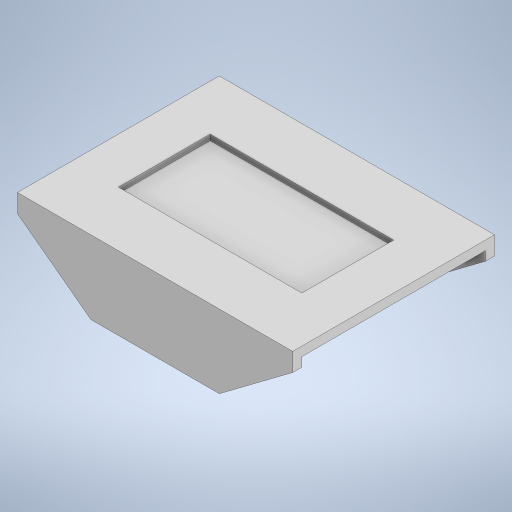
# Autodesk Inventor part: Battery Cage
Saved by Autodesk Inventor 2023 (Build 270158000, 158)
## iProperties
Created: 2022-10-27
Part Number: Battery Cage
Material: Generic
Document SubType Name: Modeling
Designer: cheng
Density: 1 g/cm^3
Appearance: Default
Author: cheng
Autodesk Inventor part; units mm, degrees
ref_plane "YZ Plane" through (0, 0, 0) normal (1, 0, 0) x (0, 1, 0)
ref_plane "XZ Plane" through (0, 0, 0) normal (0, 1, 0) x (-1, 0, 0)
ref_plane "XY Plane" through (0, 0, 0) normal (0, 0, 1) x (1, 0, 0)
sketch "Sketch1" plane through (0, 0, 0) normal (0, 1, 0) x (-1, 0, 0)
  line L0 (75, -55) -> (-75, -55)
  line L1 (-75, -55) -> (-75, 55)
  line L2 (-75, 55) -> (75, 55)
  line L3 (75, 55) -> (75, -55)
  line L4 (75, -55) -> (-75, 55) construction
  line L5 (-75, -55) -> (75, 55) construction
  point P0 (0, 0)
  dimension "d0" = 110
  dimension "d1" = 150
  constraints: 12 end point, 2 midpoint, 2 parallel, 1 horizontal, 1 perpendicular
  measures "d0" distance of L2.end L0.start
  measures "d1" distance of L0.start L0.end
extrude "Extrusion1" add sketch "Sketch1" along normal blind 40
sketch "Sketch2" plane through (75, 0, 55) normal (1, 0, 0) x (0, 0, -1)
  line L0 (55, 0) -> (55, 40)
  line L1 (105, 35) -> (5, 35)
  line L2 (5, 35) -> (5, 5)
  line L3 (5, 5) -> (105, 5)
  line L4 (105, 5) -> (105, 35)
  line L5 (105, 35) -> (5, 5) construction
  line L6 (5, 35) -> (105, 5) construction
  line L7 (0, 40) -> (110, 40) projected
  point P0 (55, 20)
  dimension "d4" = 100
  dimension "d5" = 30
  dimension "d6" = 5
  constraints: 14 end point, 3 midpoint, 2 parallel, 1 horizontal, 1 perpendicular, 1 vertical
  measures "d4" distance of L1.start L1.end
  measures "d5" distance of L3.end L1.start
  measures "d6" distance between parallel lines of L7 L1
extrude "Extrusion2" cut sketch "Sketch2" against normal through all
sketch "Sketch3" plane through (75, 0, 55) normal (1, 0, 0) x (0, 0, -1)
  line L0 (55, 0) -> (55, 5)
  line L1 (105, 5) -> (5, 5) projected
  line L2 (95, 10) -> (15, 10)
  line L3 (15, 10) -> (15, -5)
  line L4 (15, -5) -> (95, -5)
  line L5 (95, -5) -> (95, 10)
  line L6 (95, 10) -> (15, -5) construction
  line L7 (15, 10) -> (95, -5) construction
  point P0 (5, 5)
  point P1 (55, 2.5)
  point P2 (95, 5)
  point P3 (15, 5)
  point P4 (100, 15)
  point P5 (0, 15)
  point P6 (100, 15)
  dimension "d9" = 80
  constraints: 14 end point, 3 midpoint, 2 parallel, 1 horizontal, 1 perpendicular, 2 other
  measures "d9" distance of L3.end L4.end
extrude "Extrusion3" cut sketch "Sketch3" against normal through all
sketch "Sketch4" plane through (0, 40, 0) normal (0, 1, 0) x (1, 0, 0)
  line L0 (-50, 25) -> (50, 25)
  line L1 (50, 25) -> (50, -25)
  line L2 (50, -25) -> (-50, -25)
  line L3 (-50, -25) -> (-50, 25)
  line L4 (-50, 25) -> (50, -25) construction
  line L5 (50, 25) -> (-50, -25) construction
  point P0 (0, 0)
  dimension "d12" = 50
  dimension "d13" = 100
  constraints: 12 end point, 2 midpoint, 2 parallel, 1 horizontal, 1 perpendicular
  measures "d12" distance of L0.end L1.end
  measures "d13" distance of L0.start L0.end
extrude "Extrusion4" cut sketch "Sketch4" against normal blind 3
sketch "Sketch5" plane through (75, 0, -55) normal (0, 0, -1) x (-1, 0, 0)
  line L0 (0, 0) -> (150, 0) projected
  line L1 (150, 0) -> (150, 40) projected
  line L2 (0, 40) -> (150, 40) projected
  line L3 (0, 0) -> (0, 40) projected
  line L4 (150, 0) -> (0, 0) construction
  line L5 (150, 0) -> (0, 40) construction
  line L6 (0, 0) -> (0, 40) construction
  line L7 (0, 0) -> (150, 40) construction
  line L8 (75, 20) -> (75, 40) construction
  line L9 (0, 40) -> (40, 40)
  line L10 (40, 0) -> (0, 0)
  line L11 (0, 0) -> (0, 40)
  line L12 (150, 0) -> (150, 40)
  line L13 (0, 30) -> (40, 30)
  line L14 (40, 30) -> (40, 0)
  line L15 (40, 0) -> (0, 0)
  line L16 (0, 0) -> (0, 30)
  line L17 (0, 30) -> (40, 0)
  line L18 (150, 30) -> (110, 30)
  line L19 (110, 30) -> (110, 0)
  line L20 (150, 30) -> (110, 0)
  point P0 (75, 0)
  dimension "d20" = 30
  dimension "d21" = 70
  constraints: 30 end point, 4 symmetric about line, 3 parallel, 2 horizontal, 2 midpoint, 2 point on line, 1 perpendicular
  measures "d20" distance between parallel lines of L0 L13
  measures "d21" distance between parallel lines of L19 L14
extrude "Extrusion5" cut sketch "Sketch5" against normal through all contours L3 L17 L0 | L20 L1 L0
body "Solid1"
